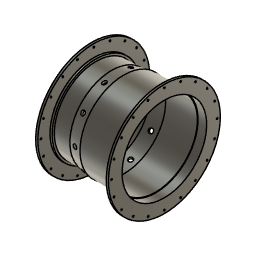
petrol_intake_case_eng_model (Autodesk Fusion 360 design; units mm, degrees)
Autodesk Fusion 360 part; units mm, degrees
sketch "Sketch1" plane through (0, 0, 0) normal (0, 1, 0) x (1, 0, 0)
  line L0 (0, -96.5) -> (0, -129.65)
  line L1 (5, -85.01) -> (5, -96.5)
  line L2 (5, -96.5) -> (0, -96.5)
  line L3 (0, -96.5) -> (0, -242.082176) construction
  line L4 (10, -101.5) -> (5, -101.5)
  line L5 (5, -101.5) -> (5, -129.65)
  line L6 (0, -129.65) -> (5, -129.65)
  line L7 (5, -96.5) -> (33.874346, -96.5) construction
  line L8 (20.83, -85.01) -> (20.83, -91.01)
  line L9 (20.83, -91.01) -> (43.83, -91.01)
  line L10 (43.83, -91.01) -> (74.98, -91.01) construction
  line L11 (43.83, -91.01) -> (74.98, -96.5)
  line L12 (74.98, -96.5) -> (148.5, -96.5)
  line L13 (168.5, -98) -> (168.5, -129.65)
  line L14 (0, -129.65) -> (2.5, -129.65)
  line L15 (0, -129.65) -> (179.710272, -129.65) construction
  line L16 (168.5, -129.65) -> (167.155938, -129.65) construction
  line L17 (5, -85.01) -> (20.83, -85.01)
  line L18 (168.5, -129.65) -> (163.5, -129.65)
  line L19 (163.5, -129.65) -> (163.5, -101.5)
  line L20 (163.5, -101.5) -> (161.589337, -101.5)
  line L21 (161.589337, -101.5) -> (74.542759, -101.5)
  line L22 (46.172996, -96.5) -> (74.542759, -101.5)
  line L23 (10, -101.5) -> (10, -96.5)
  line L24 (10, -96.5) -> (46.172996, -96.5)
  line L25 (168.5, -98) -> (148.5, -98)
  line L26 (148.5, -98) -> (148.5, -96.5)
  dimension "d2" = 129.65
  dimension "d7" = 96.5
  dimension "d8" = 85.01
  dimension "d9" = 5
  dimension "d11" = 15.83
  dimension "d12" = 6
  dimension "d13" = 23
  dimension "d14" = 31.15
  dimension "d15" = 73.52
  dimension "d16" = 96.5
  dimension "d17" = 31.15
  dimension "d19" = 129.65
  dimension "d20" = 5
  dimension "d22" = 5
  dimension "d24" = 20
  dimension "d25" = 1.5
  constraint vertical L1
  constraint horizontal L2
  constraint perpendicular L1 L7
  constraint perpendicular L8 L9
  constraint parallel L9 L10
  constraint parallel L10 L12
  constraint perpendicular L12 L13
  constraint midpoint L6 L14.end
  constraint perpendicular L3 L14
  constraint perpendicular L0 L15
  constraint perpendicular L13 L16
  constraint perpendicular L8 L17
  constraint perpendicular L13 L18
  constraint perpendicular L18 L19
  constraint perpendicular L19 L20
  constraint perpendicular L19 L21
  constraint parallel L11 L22
  constraint perpendicular L4 L23
  constraint coincident L7 L23.end
  constraint perpendicular L7 L23
  constraint perpendicular L23 L24
  constraint perpendicular L13 L25
  measures "d2" distance of origin L0.end
  measures "d7" distance of origin L2
  measures "d8" vertical distance of origin L1.start
  measures "d9" distance of L0.start L1
  measures "d11" distance of L1.start L8.start
  measures "d12" distance of L8.start L8.end
  measures "d13" distance of L8.end L9.end
  measures "d14" distance of L9.end L10.end
  measures "d15" distance of L11.end L12.end
  measures "d16" vertical distance of origin L12.end
  measures "d17" horizontal distance of L9.end L11.end
  measures "d19" vertical distance of origin L13.end
  measures "d20" distance of L13.end L18.end
  measures "d22" distance of L11 L22
  measures "d24" distance of L13 L26
  measures "d25" distance of L25.end L12.end
revolve "Revolve1" add sketch "Sketch1" angle 360 about axis through (1.75, 0, 0) along (1, 0, 0)
sketch "Sketch2" plane through (0, 0, 0) normal (-1, 0, 0) x (0, -1, 0)
  circle A0 centre (0, 0) radius 129.65
  circle A1 centre (0, 0) radius 96.5
  line L0 (0, 0) -> (0, 152.69609) construction
  circle A2 centre (0, 122.5) radius 2
  dimension "d27" = 4
  dimension "d28" = 122.5
  constraint coincident A0.centre A1.centre
  constraint vertical L0
  constraint coincident L0 A2.centre
  measures "d27" diameter of A2
  measures "d28" distance of A0.centre A2.centre
extrude "Extrude1" cut sketch "Sketch2" against normal blind 200 contours A2 picked at (0.510873, 121.750687)
pattern_circular "C-Pattern1" count 20 over 360 about axis through (1.75, 0, 0) along (1, 0, 0) of "Extrude1"
sketch "Sketch3" plane through (0, 0, 0) normal (0, 0, 1) x (1, 0, 0)
  line L0 (0, 0) -> (211.069787, 0) construction
  line L1 (74.542759, 101.5) -> (74.542759, -101.5) construction
  line L2 (46.172996, 96.5) -> (46.172996, -96.5) construction
  line L3 (46.172996, 96.5) -> (74.542759, 101.5) construction
  line L4 (60.357876, 99) -> (62.526148, 86.703116) construction
  line L5 (60.142562, 100.221105) -> (61.878251, 90.372888)
  line L6 (61.878251, 90.372888) -> (56.954143, 89.505043)
  line L7 (56.954143, 89.505043) -> (55.218454, 99.35326)
  line L8 (55.218454, 99.35326) -> (60.142562, 100.221105)
  point P0 (60.357876, 99)
  dimension "d33" = 28.807004
  dimension "d34" = 14.4035
  dimension "d35" = 10
  dimension "d36" = 5
  dimension "d37" = 10
  constraint coincident L0.start origin
  constraint horizontal L0
  constraint perpendicular L5 L6
  constraint parallel L5 L7
  constraint parallel L6 L8
  constraint perpendicular L3 L5
  measures "d35" angle of L1 L4
revolve "Revolve2" cut sketch "Sketch3" angle 360 about axis through (60.142562, 100.221105, 0) along (0.173569, -0.984822, 0)
pattern_circular "C-Pattern2" count 10 over 360 about axis through (1.75, 0, 0) along (1, 0, 0) of "Revolve2"
equation "d16 = 101.5 mm - 5 mm"
equation "d34 = ( 28.807 / 2 ) * 1 mm"
